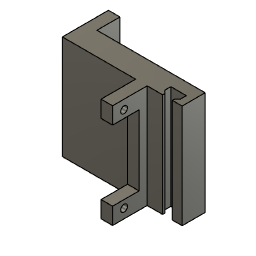
FrameV1 (Autodesk Fusion 360 design; units mm, degrees)
Autodesk Fusion 360 part; units mm, degrees
sketch "Sketch1" plane through (0, 0, 0) normal (0, 1, 0) x (1, 0, 0)
  line L0 (0, 0) -> (52, 0)
  line L1 (52, 0) -> (52, -10)
  line L2 (52, -10) -> (0, -10)
  line L3 (0, -10) -> (0, 0)
  line L4 (0, 0) -> (5, 0)
  line L5 (5, 0) -> (5, 10)
  line L6 (5, 10) -> (0, 10)
  line L7 (0, 10) -> (0, 0)
  dimension "d1" = 52
  dimension "d2" = 10
  dimension "d3" = 5
  dimension "d4" = 10
  constraint horizontal L0
  constraint vertical L1
  constraint horizontal L2
  constraint vertical L3
  constraint coincident L0.start L3.end
  constraint horizontal L4
  constraint vertical L5
  constraint horizontal L6
  constraint vertical L7
  measures "d1" distance of L0.start L0.end
  measures "d2" distance of L0.start L2.end
  measures "d3" distance of L0.start L4.end
  measures "d4" distance of L0.start L6.end
extrude "Extrude1" add sketch "Sketch1" along normal blind 45
sketch "Sketch2" plane through (0, 45, 0) normal (0, 1, 0) x (-1, 0, 0)
  line L0 (-5, 0) -> (-5, -10)
  line L1 (-5, -10) -> (0, -10)
  line L2 (0, -10) -> (0, 10)
  line L3 (0, 10) -> (-52, 10)
  line L4 (-52, 10) -> (-52, 0)
  line L5 (-52, 0) -> (-5, 0)
  line L6 (-49, 7.834) -> (-42.269, 7.834)
  line L7 (-42.269, 7.834) -> (-42.269, 5.174)
  line L8 (-42.269, 5.174) -> (-49, 5.174)
  line L9 (-49, 5.174) -> (-49, 7.834)
  line L10 (-49, 7.834) -> (-42.269, 5.174) construction
  line L11 (-42.269, 7.834) -> (-49, 5.174) construction
  line L12 (-47.7345, 10) -> (-43.5345, 10)
  line L13 (-43.5345, 10) -> (-43.5345, 9)
  line L14 (-43.5345, 9) -> (-47.7345, 9)
  line L15 (-47.7345, 9) -> (-47.7345, 10)
  line L16 (-47.7345, 10) -> (-43.5345, 9) construction
  line L17 (-43.5345, 10) -> (-47.7345, 9) construction
  line L18 (-47.7345, 9) -> (-49, 7.834)
  line L19 (-43.5345, 9) -> (-42.269, 7.834)
  line L20 (-45.6345, 6.504) -> (-45.6345, 9.5)
  point P0 (-45.6345, 6.504)
  point P1 (-45.6345, 9.5)
  dimension "rail_upper_part_depth" = 1
  dimension "rail_upper_part_width" = 4.2
  dimension "rail_depth" = 4.826
  dimension "rail_base_depth" = 2.66
  dimension "rail_edge_position" = 3
  dimension "rail_base_width" = 6.731
  constraint horizontal L6
  constraint perpendicular L6 L7
  constraint parallel L6 L8
  constraint parallel L7 L9
  constraint coincident L10 P0
  constraint coincident L11 P0
  constraint horizontal L12
  constraint perpendicular L12 L13
  constraint parallel L12 L14
  constraint parallel L13 L15
  constraint coincident L16 P1
  constraint coincident L17 P1
  constraint coincident L3 L12.start
  constraint coincident P0 L20.start
  constraint coincident P1 L20.end
  constraint perpendicular L14 L20
  measures "rail_upper_part_depth" distance of L12 L14
  measures "rail_upper_part_width" distance of L13 L15
  measures "rail_depth" distance of L3 L8
  measures "rail_base_depth" distance of L6 L8
  measures "rail_edge_position" distance of L4 L9
  measures "rail_base_width" distance of L7 L9
extrude "Extrude2" cut sketch "Sketch2" against normal up to surface (45 mm away) contours L3 L12 L13 L14 L15 | L6 L14 L18 L20 | L6 L14 L19 L20 | L6 L7 L8 L9
ref_plane "WorkPlane1" through (36.8045, 22.5, 9.5) normal (1, 0, 0) x (0, 0, 1)
sketch "Sketch3" plane through (36.8045, 22.5, 9.5) normal (1, 0, 0) x (0, 0, -1)
  line L0 (-0.5, -22.5) -> (-15.5, -22.5)
  line L1 (-15.5, -22.5) -> (-15.5, 22.5)
  line L2 (-15.5, 22.5) -> (-0.5, 22.5)
  line L3 (-0.5, 22.5) -> (-0.5, -22.5)
  line L4 (-0.5, 22.5) -> (9.5, 22.5)
  line L5 (9.5, -22.5) -> (-0.5, -22.5)
  line L6 (-0.5, -22.5) -> (-0.5, 22.5)
  line L7 (-15.5, -15.25) -> (-4, -15.25)
  line L8 (-4, -15.25) -> (-4, 15.25)
  line L9 (-4, 15.25) -> (-15.5, 15.25)
  line L10 (-15.5, 15.25) -> (-15.5, -15.25)
  line L11 (-15.5, -15.25) -> (-4, 15.25) construction
  line L12 (-4, -15.25) -> (-15.5, 15.25) construction
  circle A0 centre (-10.5, -18.5) radius 1.5
  line L13 (-15.5, 0) -> (-4, 0)
  circle A1 centre (-10.5, 18.5) radius 1.5
  point P0 (-9.75, 0)
  dimension "moto_holder_frae_length" = 15
  dimension "motor_width_space" = 30.5
  dimension "d22" = 22.5
  dimension "d23" = 37
  dimension "d25" = 3
  dimension "holes_from_surface2" = 10
  dimension "d27" = 3.5
  constraint horizontal L0
  constraint vertical L1
  constraint horizontal L2
  constraint vertical L3
  constraint collinear L2 L4
  constraint collinear L0 L5
  constraint collinear L3 L6
  constraint horizontal L7
  constraint perpendicular L7 L8
  constraint parallel L7 L9
  constraint parallel L8 L10
  constraint coincident L11 P0
  constraint coincident L12 P0
  constraint coincident L1 L7.start
  constraint midpoint L10 L13.start
  constraint midpoint L8 L13.end
  constraint symmetric A0 L13 A1
  measures "moto_holder_frae_length" distance of L1 L3
  measures "motor_width_space" distance of L7 L9
  measures "d22" distance of L2 P0
  measures "d25" diameter of A0
  measures "holes_from_surface2" distance of L3 A1.centre
  measures "d27" distance of L3 L8
extrude "Extrude3" add sketch "Sketch3" against normal blind 5 contours L0 L1 L2 L3 L6 L7 L8 L9
sketch "Sketch4" plane through (5, 0, 0) normal (1, 0, 0) x (0, 0, -1)
  line L0 (0, 0) -> (10, 0)
  line L1 (10, 0) -> (10, 45)
  line L2 (10, 45) -> (0, 45)
  line L3 (0, 45) -> (0, 0)
  line L4 (10, 22.5) -> (0, 22.5)
  circle A0 centre (5, 37.5) radius 1.5
  circle A1 centre (5, 7.5) radius 1.5
  dimension "d30" = 3
  dimension "d31" = 5
  dimension "d32" = 30
  constraint midpoint L1 L4.start
  constraint midpoint L3 L4.end
  constraint symmetric L4 A0 A1
  measures "d30" diameter of A0
  measures "d31" distance of L3 A0.centre
  measures "d32" distance of A0.centre A1.centre
extrude "Extrude4" cut sketch "Sketch4" against normal up to surface (5 mm away) contours A0 | A1
equation "d5 = 45 mm"
equation "motor_holder_from_rail_edge = -6.73 mm"
equation "d22 = d5 / 2"
